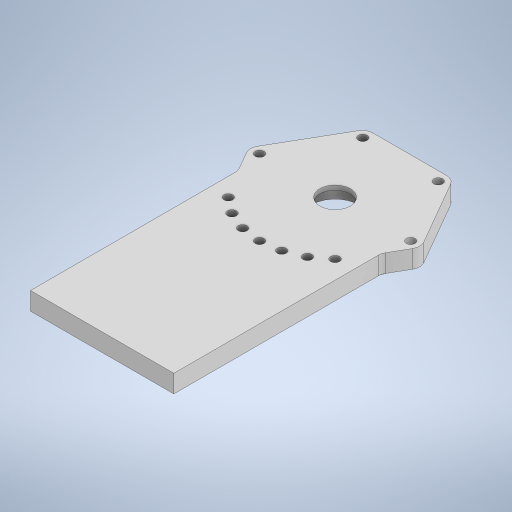
# Autodesk Inventor part: ZadKriska
Saved by Autodesk Inventor 2024 (Build 280153000, 153)
## iProperties
Created: 2023-08-25
Part Number: ZadKriska
Material: Generic
Document SubType Name: Modeling
Designer: KirikDK
Density: 1 g/cm^3
Appearance: Default
Author: KirikDK
Autodesk Inventor part; units mm, degrees
ref_plane "YZ Plane" through (0, 0, 0) normal (1, 0, 0) x (0, 1, 0)
ref_plane "XZ Plane" through (0, 0, 0) normal (0, 1, 0) x (-1, 0, 0)
ref_plane "XY Plane" through (0, 0, 0) normal (0, 0, 1) x (1, 0, 0)
sketch "Sketch1" plane through (0, 0, 0) normal (0, 1, 0) x (-1, 0, 0)
  line L0 (83.678612, 197.794487) -> (-76.321388, 197.794487)
  line L1 (-76.321388, 197.794487) -> (-76.321388, -52.205513)
  line L2 (-76.321388, -52.205513) -> (83.678612, -52.205513)
  line L3 (83.678612, -52.205513) -> (83.678612, 197.794487)
  circle A0 centre (3.678612, -62.205513) radius 80
  line L4 (83.678612, -52.205513) -> (83.678612, -62.205513)
  line L5 (-76.321388, -52.205513) -> (-76.321388, -62.205513)
  circle A1 centre (3.678612, -62.205513) radius 26
  circle A2 centre (3.678612, -62.205513) radius 40
  point P0 (0, 0)
  point P1 (59.392898, -23.634084)
  point P2 (-75.693927, -52.205513)
  point P3 (83.051152, -52.205513)
  dimension "d0" = 250
  dimension "d1" = 160
  dimension "d2" = 160
  dimension "d3" = 10
  dimension "d4" = 52
  dimension "d5" = 80
  constraints: 12 end point, 3 centre point, 2 coincident, 2 parallel, 2 point on circle, 1 horizontal, 1 perpendicular, 1 tangent, 1 vertical
  measures "d0" distance of L2.end L0.start
  measures "d1" distance of L0.start L0.end
  measures "d2" diameter of A0
  measures "d3" distance from line of A0.centre L2
  measures "d4" diameter of A1
  measures "d5" diameter of A2
extrude "Extrusion1" add sketch "Sketch1" along normal blind 20 contours L3 L2 A0 L1 L0 | L4 A0 L2 | L2 A0 L5 | A0 L2 A2 | L2 A2 A0 | A2 L2 A1 | L2 A1 A2
sketch "Sketch2" plane through (0, 20, 0) normal (0, 1, 0) x (1, 0, 0)
  circle A0 centre (-3.678612, 62.205513) radius 26
  circle A1 centre (-3.678612, 62.205513) radius 26
  circle A2 centre (-3.678612, 62.205513) radius 17
  point P0 (0, 0)
  dimension "d8" = 34
  constraints: 2 centre point, 2 coincident
  measures "d8" diameter of A2
extrude "Extrusion2" add sketch "Sketch2" against normal blind 5
sketch "Sketch3" plane through (0, 0, 0) normal (0, -1, 0) x (1, 0, 0)
  circle A0 centre (-3.678612, -62.205513) radius 75
  circle A1 centre (-3.678612, -62.205513) radius 75
  line L0 (92.607102, -62.205513) -> (44.464245, -145.591387)
  line L1 (44.464245, -145.591387) -> (-51.821469, -145.591387)
  line L2 (-51.821469, -145.591387) -> (-99.964327, -62.205513)
  line L3 (-99.964327, -62.205513) -> (-51.821469, 21.180362)
  line L4 (-51.821469, 21.180362) -> (44.464245, 21.180362)
  line L5 (44.464245, 21.180362) -> (92.607102, -62.205513)
  line L6 (80.607102, -62.205513) -> (38.464245, -135.199083)
  line L7 (38.464245, -135.199083) -> (-45.821469, -135.199083)
  line L8 (-45.821469, -135.199083) -> (-87.964327, -62.205513)
  line L9 (-87.964327, -62.205513) -> (-45.821469, 10.788057)
  line L10 (-45.821469, 10.788057) -> (38.464245, 10.788057)
  line L11 (38.464245, 10.788057) -> (80.607102, -62.205513)
  circle A2 centre (80.607102, -62.205513) radius 5
  circle A3 centre (38.464245, 10.788057) radius 5
  circle A4 centre (-45.821469, 10.788057) radius 5
  circle A5 centre (-87.964327, -62.205513) radius 5
  circle A6 centre (-45.821469, -135.199083) radius 5
  circle A7 centre (38.464245, -135.199083) radius 5
  circle A8 centre (-3.678612, -62.205513) radius 26
  circle A9 centre (-3.678612, -62.205513) radius 0.853538
  point P0 (0, 0)
  point P1 (-59.392898, -100.776941)
  point P2 (-3.678612, -62.205513)
  dimension "d13" = 360
  constraints: 24 end point, 9 centre point, 5 coincident, 39 other
sketch "Sketch4" plane through (0, 0, 0) normal (0, -1, 0) x (1, 0, 0)
  circle A0 centre (-45.821469, -135.199083) radius 5
  line L0 (-45.821469, -135.199083) -> (-87.964327, -62.205513)
  line L1 (-51.821469, -145.591387) -> (-99.964327, -62.205513)
  circle A1 centre (-87.964327, -62.205513) radius 5
  circle A2 centre (-45.821469, 10.788057) radius 5
  line L2 (-87.964327, -62.205513) -> (-45.821469, 10.788057)
  line L3 (-99.964327, -62.205513) -> (-51.821469, 21.180362)
  line L4 (38.464245, -135.199083) -> (-45.821469, -135.199083)
  circle A3 centre (38.464245, -135.199083) radius 5
  line L5 (44.464245, -145.591387) -> (-51.821469, -145.591387)
  line L6 (80.607102, -62.205513) -> (38.464245, -135.199083)
  line L7 (92.607102, -62.205513) -> (44.464245, -145.591387)
  circle A4 centre (-3.678612, -62.205513) radius 75
  circle A5 centre (-3.678612, -62.205513) radius 75
  line L8 (-45.821469, 10.788057) -> (38.464245, 10.788057)
  line L9 (-51.821469, 21.180362) -> (44.464245, 21.180362)
  circle A6 centre (80.607102, -62.205513) radius 5
  circle A7 centre (38.464245, 10.788057) radius 5
  line L10 (38.464245, 10.788057) -> (80.607102, -62.205513)
  line L11 (44.464245, 21.180362) -> (92.607102, -62.205513)
  circle A8 centre (-3.678612, -62.205513) radius 26
  circle A9 centre (-3.678612, -62.205513) radius 17
  circle A10 centre (-3.678612, -62.205513) radius 2.321388
  point P0 (0, 0)
  point P1 (0, 0)
  point P2 (-59.392898, -100.776941)
  dimension "d18" = 360
  constraints: 24 end point, 10 centre point, 5 coincident, 39 other
extrude "Extrusion3" cut sketch "Sketch3" against normal blind 22 contours A2 L6 L11 | L11 L6 A2 | A3 L10 L11 | L11 L10 A3 | A7 L7 L6 | L6 L7 A7 | A4 L9 L10 | L10 L9 A4 | A6 L8 L7 | L7 L8 A6 | A5 L8 L9 | L9 L8 A5
extrude "Extrusion4" add sketch "Sketch4" against normal blind 20 contours A0 L0 A4 L4 | A4 L6 A3 L4 | L0 A1 L2 A4 | A4 L10 A6 L6 | L2 A2 L8 A4 | L8 A7 L10 A4 | L1 L3 L9 L11 L7 L5
sketch "Sketch5" plane through (0, 0, 0) normal (0, -1, 0) x (1, 0, 0)
  circle A0 centre (-3.678612, -62.205513) radius 17
  circle A1 centre (-3.678612, -62.205513) radius 79.285714
  circle A2 centre (80.607102, -62.205513) radius 5
  circle A3 centre (-3.678612, -62.205513) radius 75
  point P0 (0, 0)
  dimension "d21" = 150
  constraints: 2 centre point, 2 coincident, 1 tangent
  measures "d21" diameter of A3
extrude "Extrusion5" add sketch "Sketch5" along normal blind 5 contours A1
fillet "Fillet1" radius 12 6 edges at (-83.6786, 10, -33.9978) (-99.9643, 10, -62.2055) (-51.8215, 10, -145.5914) (44.4642, 10, -145.5914) (92.6071, 10, -62.2055) (76.3214, 10, -33.9978)
sketch "Sketch6" plane through (0, 0, 0) normal (0, -1, 0) x (1, 0, 0)
  arc A0 (89.143, -68.205513) -> (89.143, -56.205513) centre (78.750696, -62.205513) ccw
  line L0 (89.143, -56.205513) -> (77.929083, -36.782438)
  arc A1 (76.321388, -30.782438) -> (77.929083, -36.782438) centre (88.321388, -30.782438) ccw
  line L1 (76.321388, 197.794487) -> (76.321388, -30.782438)
  line L2 (-83.678612, 197.794487) -> (76.321388, 197.794487)
  line L3 (-83.678612, -30.782438) -> (-83.678612, 197.794487)
  arc A2 (-85.286307, -36.782438) -> (-83.678612, -30.782438) centre (-95.678612, -30.782438) ccw
  line L4 (-85.286307, -36.782438) -> (-96.500225, -56.205513)
  arc A3 (-96.500225, -56.205513) -> (-96.500225, -68.205513) centre (-86.10792, -62.205513) ccw
  line L5 (-96.500225, -68.205513) -> (-55.285571, -139.591387)
  arc A4 (-55.285571, -139.591387) -> (-44.893266, -145.591387) centre (-44.893266, -133.591387) ccw
  line L6 (-44.893266, -145.591387) -> (37.536042, -145.591387)
  arc A5 (37.536042, -145.591387) -> (47.928346, -139.591387) centre (37.536042, -133.591387) ccw
  line L7 (47.928346, -139.591387) -> (89.143, -68.205513)
  circle A6 centre (-87.964327, -62.205513) radius 5
  arc A7 (-43.321469, 6.45793) -> (-82.964327, -62.205513) centre (-3.678612, -62.205513) ccw
  circle A8 centre (-45.821469, 10.788057) radius 5
  arc A9 (35.964245, 6.45793) -> (-43.321469, 6.45793) centre (-3.678612, -62.205513) ccw
  circle A10 centre (38.464245, 10.788057) radius 5
  arc A11 (75.607102, -62.205513) -> (35.964245, 6.45793) centre (-3.678612, -62.205513) ccw
  circle A12 centre (80.607102, -62.205513) radius 5
  arc A13 (35.964245, -130.868956) -> (75.607102, -62.205513) centre (-3.678612, -62.205513) ccw
  circle A14 centre (38.464245, -135.199083) radius 5
  arc A15 (-43.321469, -130.868956) -> (35.964245, -130.868956) centre (-3.678612, -62.205513) ccw
  circle A16 centre (-45.821469, -135.199083) radius 5
  arc A17 (-82.964327, -62.205513) -> (-43.321469, -130.868956) centre (-3.678612, -62.205513) ccw
  arc A18 (56.321388, -30.782438) -> (60.608575, -46.782438) centre (88.321388, -30.782438) ccw
  line L8 (60.608575, -46.782438) -> (69.513091, -62.205513)
  line L9 (69.513091, -62.205513) -> (32.917239, -125.591387)
  line L10 (32.917239, -125.591387) -> (-40.274464, -125.591387)
  line L11 (-40.274464, -125.591387) -> (-76.870316, -62.205513)
  line L12 (-76.870316, -62.205513) -> (-67.965799, -46.782438)
  arc A19 (-67.965799, -46.782438) -> (-63.678612, -30.782438) centre (-95.678612, -30.782438) ccw
  line L13 (-63.678612, -30.782438) -> (-63.678612, 177.794487)
  line L14 (-63.678612, 177.794487) -> (56.321388, 177.794487)
  line L15 (56.321388, 177.794487) -> (56.321388, -30.782438)
  arc A20 (-53.321469, 23.778438) -> (-102.964327, -62.205513) centre (-3.678612, -62.205513) ccw
  arc A21 (-102.964327, -62.205513) -> (-53.321469, -148.189464) centre (-3.678612, -62.205513) ccw
  arc A22 (-53.321469, -148.189464) -> (45.964245, -148.189464) centre (-3.678612, -62.205513) ccw
  arc A23 (45.964245, -148.189464) -> (95.607102, -62.205513) centre (-3.678612, -62.205513) ccw
  arc A24 (95.607102, -62.205513) -> (45.964245, 23.778438) centre (-3.678612, -62.205513) ccw
  arc A25 (45.964245, 23.778438) -> (-53.321469, 23.778438) centre (-3.678612, -62.205513) ccw
  point P0 (0, 0)
  point P1 (-63.678612, 16.899816)
  point P2 (56.321388, 16.899816)
  dimension "d25" = 20
  dimension "d26" = 20
  constraints: 16 end point, 16 point on circle, 8 centre point, 2 horizontal alignment, 18 other
  measures "d25" distance between parallel lines of L1 L15
  measures "d26" radial gap between concentric circles of A9 A25
sketch "Sketch6 outline for Extrusion6" plane through (0, 0, 0) normal (0, -1, 0) x (1, 0, 0)
  line L0 (56.321388, 177.794487) -> (-63.678612, 177.794487)
  line L1 (56.321388, 16.899816) -> (56.321388, 177.794487)
  arc A0 (45.964245, 23.778438) -> (56.321388, 16.899816) centre (-3.678612, -62.205513) cw
  arc A1 (-53.321469, 23.778438) -> (45.964245, 23.778438) centre (-3.678612, -62.205513) cw
  arc A2 (-63.678612, 16.899816) -> (-53.321469, 23.778438) centre (-3.678612, -62.205513) cw
  line L2 (-63.678612, 177.794487) -> (-63.678612, 16.899816)
extrude "Extrusion6" cut sketch "Sketch6 outline for Extrusion6" against normal blind 12
sketch "Sketch7" plane through (0, 0, 0) normal (0, -1, 0) x (1, 0, 0)
  circle A0 centre (-3.678612, 22.080487) radius 5
  circle A1 centre (-3.678612, -62.205513) radius 17
  circle A2 centre (-25.493434, 19.208511) radius 5
  circle A3 centre (-45.821612, 10.788304) radius 5
  circle A4 centre (-63.277814, -2.606311) radius 5
  circle A5 centre (-76.672429, -20.062513) radius 5
  circle A6 centre (-85.092637, -40.390691) radius 5
  circle A7 centre (-87.964612, -62.205513) radius 5
  circle A8 centre (-85.092637, -84.020335) radius 5
  circle A9 centre (-76.672429, -104.348513) radius 5
  circle A10 centre (-63.277814, -121.804715) radius 5
  circle A11 centre (-45.821612, -135.19933) radius 5
  circle A12 centre (-25.493434, -143.619537) radius 5
  circle A13 centre (-3.678612, -146.491513) radius 5
  circle A14 centre (18.13621, -143.619537) radius 5
  circle A15 centre (38.464388, -135.19933) radius 5
  circle A16 centre (55.92059, -121.804715) radius 5
  circle A17 centre (69.315205, -104.348513) radius 5
  circle A18 centre (77.735412, -84.020335) radius 5
  circle A19 centre (80.607388, -62.205513) radius 5
  circle A20 centre (77.735412, -40.390691) radius 5
  circle A21 centre (69.315205, -20.062513) radius 5
  circle A22 centre (55.92059, -2.606311) radius 5
  circle A23 centre (38.464388, 10.788304) radius 5
  circle A24 centre (18.13621, 19.208511) radius 5
  point P0 (0, 0)
  dimension "d29" = 84.286
  dimension "d30" = 10
  dimension "d33" = 360
  constraints: 24 centre point, 49 other
  measures "d29" distance of A1.centre A0.centre
  measures "d30" diameter of A0
extrude "Extrusion7" cut sketch "Sketch7" against normal blind 39 contours A0 | A2 | A4 | A5 | A21 | A22 | A24
sketch "Sketch8" plane through (0, 20, 0) normal (0, 1, 0) x (1, 0, 0)
  circle A0 centre (69.315205, 20.062513) radius 5
  circle A1 centre (-76.672429, 20.062513) radius 5
  point P0 (0, 0)
extrude "Extrusion8" add sketch "Sketch8" against normal blind 20
body "Solid1"
